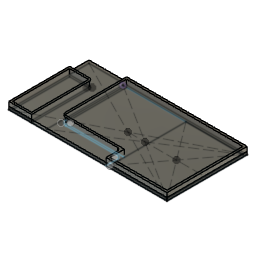
RPM Holder (Autodesk Fusion 360 design; units mm, degrees)
Autodesk Fusion 360 part; units mm, degrees
sketch "Sketch2" plane through (0, 0, 0) normal (0, 0, 1) x (1, 0, 0)
  line L0 (0, 0) -> (127, 0)
  line L1 (127, 0) -> (127, -80.5)
  line L2 (127, -80.5) -> (0, -80.5)
  line L3 (0, -80.5) -> (0, 0)
  line L4 (66.75, -0.25) -> (126.75, -0.25)
  line L5 (126.75, -0.25) -> (126.75, -80.25)
  line L6 (126.75, -80.25) -> (66.75, -80.25)
  line L7 (66.75, -80.25) -> (66.75, -72.25)
  line L8 (66.75, -0.25) -> (3.9, -0.25)
  line L9 (3.9, -0.25) -> (3.9, -65.25)
  line L10 (3.9, -65.25) -> (65.75, -65.25)
  line L11 (66.75, -65.25) -> (66.75, -0.25)
  line L12 (-37.85, 2) -> (129, 2)
  line L13 (129, 2) -> (129, -82.5)
  line L14 (129, -82.5) -> (-37.85, -82.5)
  line L15 (-37.85, -82.5) -> (-37.85, 2)
  line L16 (127, 0) -> (0, -80.5) construction
  line L17 (0, 0) -> (127, -80.5) construction
  line L18 (-37.85, 2) -> (129, -82.5) construction
  line L19 (129, 2) -> (-37.85, -82.5) construction
  line L20 (45.575, -40.25) -> (129, -40.25) construction
  line L21 (126.75, -0.25) -> (66.75, -80.25) construction
  line L22 (66.75, -0.25) -> (126.75, -80.25) construction
  line L23 (66.75, -65.25) -> (66.75, -70.25)
  line L24 (1.9, -0.25) -> (1.9, -62.25)
  line L25 (3.9, -0.25) -> (1.9, -0.25) construction
  line L26 (6.9, -67.25) -> (61.75, -67.25)
  line L27 (65.75, -65.25) -> (66.75, -65.25)
  line L28 (66.75, -70.25) -> (66.75, -72.25)
  arc A0 (1.9, -62.25) -> (6.9, -67.25) centre (6.9, -62.25) ccw
  line L29 (-15.85, -20.5) -> (-35.85, -20.5)
  line L30 (-35.85, -20.5) -> (-35.85, -80.5)
  line L31 (-35.85, -80.5) -> (-15.85, -80.5)
  line L32 (-15.85, -80.5) -> (-15.85, -20.5)
  line L33 (-13.85, -80.5) -> (-37.85, -80.5)
  line L34 (-37.85, -18.5) -> (-16.85, -18.5)
  line L35 (-13.85, -21.5) -> (-13.85, -80.5)
  line L36 (1.9, -0.25) -> (1.9, 2)
  line L37 (-13.85, -80.5) -> (-13.85, -82.5)
  line L38 (66.75, -80.25) -> (66.75, -80.25)
  line L39 (61.75, -67.25) -> (61.75, -67.25)
  line L40 (64.75, -78.25) -> (64.75, -70.25)
  arc A1 (64.75, -70.25) -> (61.75, -67.25) centre (61.75, -70.25) ccw
  line L41 (64.75, -78.25) -> (64.75, -80.25)
  line L42 (64.75, -80.25) -> (64.75, -82.5)
  arc A2 (-13.85, -21.5) -> (-16.85, -18.5) centre (-16.85, -21.5) ccw
  point P0 (63.5, -40.25)
  point P1 (45.575, -40.25)
  point P2 (96.75, -40.25)
  point P3 (1.9, -67.25)
  point P4 (-13.85, -18.5)
  dimension "d4" = 127
  dimension "d5" = 80.5
  dimension "d6" = 60
  dimension "d7" = 80
  dimension "d12" = 62.85
  dimension "d13" = 65
  dimension "d17" = 166.85
  dimension "d18" = 84.5
  dimension "d23" = 0.25
  dimension "d24" = 2
  dimension "d25" = 2
  dimension "d26" = 2
  dimension "d28" = 67
  dimension "d31" = 2
  dimension "d33" = 5
  dimension "d36" = 20
  dimension "d37" = 60
  dimension "d39" = 19.75
  dimension "d41" = 2
  dimension "d42" = 24
  dimension "d45" = 2
  dimension "d46" = 3
  dimension "d50" = 3
  dimension "d51" = 2
  constraint horizontal L0
  constraint vertical L1
  constraint horizontal L2
  constraint vertical L3
  constraint coincident L0.start L3.end
  constraint horizontal L4
  constraint vertical L5
  constraint horizontal L6
  constraint vertical L7
  constraint horizontal L8
  constraint vertical L9
  constraint horizontal L10
  constraint vertical L11
  constraint horizontal L12
  constraint vertical L13
  constraint horizontal L14
  constraint vertical L15
  constraint midpoint L16 P0
  constraint midpoint L18 P1
  constraint coincident P1 L20.start
  constraint midpoint L13 L20.end
  constraint coincident P0 L20
  constraint midpoint L21 P2
  constraint coincident L20 P2
  constraint collinear L7 L11
  constraint coincident L4.start L7
  constraint coincident L11.start L10
  constraint parallel L9 L24
  constraint perpendicular L24 L25
  constraint perpendicular L23 L26
  constraint coincident L7 L23.end
  constraint perpendicular L11 L27
  constraint coincident P3 L24
  constraint coincident P3 L26
  constraint tangent L24 A0
  constraint tangent L26 A0
  constraint horizontal L29
  constraint vertical L30
  constraint horizontal L31
  constraint vertical L32
  constraint coincident L15 L33.end
  constraint perpendicular L15 L33
  constraint collinear L31 L33
  constraint coincident L15 L34.start
  constraint perpendicular L15 L34
  constraint perpendicular L33 L35
  constraint coincident L12 L36.end
  constraint perpendicular L12 L36
  constraint coincident L14 L37.end
  constraint perpendicular L14 L37
  constraint tangent L40 A1
  constraint parallel L40 L41
  constraint coincident L14 L42.end
  constraint perpendicular L14 L42
  constraint coincident P4 L34
  constraint coincident P4 L35
  constraint tangent L34 A2
  constraint tangent L35 A2
  measures "d4" distance of L0.start L0.end
  measures "d5" distance of L0.start L2.end
  measures "d6" distance of L4.start L4.end
  measures "d7" distance of L4.start L6.end
  measures "d12" distance of L4.start L8.end
  measures "d13" distance of L8.end L9.end
  measures "d17" distance of L12.start L12.end
  measures "d18" distance of L12.start L14.end
  measures "d23" distance of L1 L5
  measures "d24" distance of L1 L13
  measures "d25" distance of L0 L12
  measures "d26" distance of L2 L14
  measures "d28" distance of L24.start P3
  measures "d31" distance of L9 L24
  measures "d33" radius of A0
  measures "d36" distance of L29.start L29.end
  measures "d37" distance of L29.start L31.end
  measures "d39" distance of L9 L32
  measures "d41" distance of L29 L34
  measures "d42" distance of L34.start P4
  measures "d45" distance of L6.end L41.end
  measures "d46" radius of A1
  measures "d50" radius of A2
  measures "d51" distance of L14 L33
extrude "Extrude1" add sketch "Sketch2" along normal blind 3 contours L0 L2 L3 L12 L14 L15 L34 L35 L36 L37 L42 A2 | L0 L2 L3 L24 L26 A0 L36 L40 A1 L41 L42 | L0 L1 L2 L12 L13 L14 L36 L42 | L0 L1 L2 L24 L26 A0 L36 L40 A1 L41 L42 | L15 L29 L30 L32 L33 L34 L35 A2 | L14 L15 L31 L33 L37 | L29 L30 L31 L32 L33 | L8 L9 L10 L11 L27 | L4 L5 L6 L7 L11 L23 L28 makes body 1
extrude "Extrude2" add sketch "Sketch2" along normal blind 7.5 separate body contours L0 L1 L2 L12 L13 L14 L36 L42 | L0 L1 L2 L24 L26 A0 L36 L40 A1 L41 L42 | L15 L29 L30 L32 L33 L34 L35 A2 | L14 L15 L31 L33 L37 makes body 2 at (44.2667, 2, 2.5) makes body 3 at (-37.85, -61.1667, 2.5)
equation "d28 = d13 + 2 mm"
equation "d42 = d36 + 4 mm"
